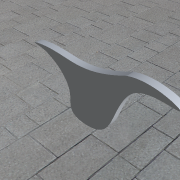
# Autodesk Inventor part: Frame_Generator
Saved by Autodesk Inventor 2014 (Build 180170000, 170)
## iProperties
Created: 2015-03-25
Part Number: Frame_Generator
Material: Générique
Document SubType Name: Modeling
Designer: Yann
Density: 1 g/cm^3
Appearance: Par défaut
Author: Yann
Autodesk Inventor part; units mm, degrees
ref_plane "YZ Plane" through (0, 0, 0) normal (1, 0, 0) x (0, 1, 0)
ref_plane "XZ Plane" through (0, 0, 0) normal (0, 1, 0) x (-1, 0, 0)
ref_plane "XY Plane" through (0, 0, 0) normal (0, 0, 1) x (1, 0, 0)
sketch "Esquisse1" plane through (0, 0, 0) normal (0, 1, 0) x (-1, 0, 0)
  line L0 (-340, 901.3144) -> (1610, 901.3144) construction
  line L1 (1610, 901.3144) -> (1610, -357) construction
  line L2 (1610, -357) -> (-340, -357) construction
  line L3 (-340, -357) -> (-340, 901.3144) construction
  line L4 (0, -14) -> (0, 14) construction
  line L5 (0, -14) -> (0, 14)
  line L6 (-730, 0) -> (2000, 0) construction
  circle A0 centre (0, 0) radius 279 construction
  line L7 (337.3918, 627.9737) -> (689.2363, 464.4505) construction
  line L8 (689.2363, 464.4505) -> (938.28, 570.241) construction
  line L9 (938.28, 570.241) -> (1415.137, 504.3626) construction
  line L10 (1415.137, 504.3626) -> (1156.5045, 515.069) construction
  line L11 (1156.5045, 515.069) -> (1075.5744, 464.4505) construction
  line L12 (1075.5744, 464.4505) -> (964.8076, 415.377) construction
  line L13 (964.8076, 415.377) -> (840.1102, 262.9378) construction
  line L14 (840.1102, 262.9378) -> (874.529, 122.2641) construction
  line L15 (874.529, 122.2641) -> (852.893, 0) construction
  line L16 (852.893, 0) -> (570.9128, 0) construction
  line L17 (570.9128, 0) -> (461.4564, 118.9329) construction
  line L18 (461.4564, 118.9329) -> (421.0876, 240.9099) construction
  line L19 (421.0876, 240.9099) -> (379.7116, 365.9298) construction
  line L20 (379.7116, 365.9298) -> (301.7206, 535.5968) construction
  line L21 (301.7206, 535.5968) -> (171.7383, 570.0881) construction
  line L22 (171.7383, 570.0881) -> (48.4505, 569.2162) construction
  line L23 (48.4505, 569.2162) -> (-58.2695, 547.8034) construction
  line L24 (-58.2695, 547.8034) -> (-58.2695, 582.2557) construction
  line L25 (-58.2695, 582.2557) -> (197.2095, 665.9211) construction
  line L26 (197.2095, 665.9211) -> (337.3918, 627.9737) construction
  spline S0 degree 4 poles (337.3918, 627.9737) (689.2363, 464.4505) (938.28, 570.241) (1415.137, 504.3626) (1156.5045, 515.069) (1075.5744, 464.4505) (964.8076, 415.377) (840.1102, 262.9378) (874.529, 122.2641) (852.893, 0) (570.9128, 0) (461.4564, 118.9329) (421.0876, 240.9099) (379.7116, 365.9298) (301.7206, 535.5968) (171.7383, 570.0881) (48.4505, 569.2162) (-58.2695, 547.8034) (-58.2695, 582.2557) (197.2095, 665.9211) (337.3918, 627.9737) knots 1 1 1 1 1 2 3 4 5 6 7 8 9 10 11 12 13 14 15 16 17 18 18 18 18 18
  dimension "d23" = 357
  dimension "d24" = 340
  dimension "d26" = 1950
  dimension "d27" = 558
  constraints: 4 end point, 2 point on line, 2 vertical, 1 centre point, 1 coincident, 1 horizontal, 8 other
  measures "d23" distance between parallel lines of L6 L2
  measures "d24" distance between parallel lines of L4 L3
  measures "d26" distance of L0.start L0.end
  measures "d27" diameter of A0
extrude "Extrusion1" add sketch "Esquisse1" along normal mid plane 66
